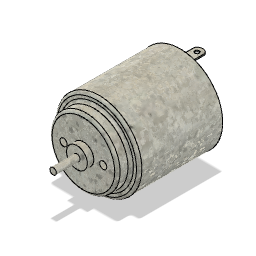
moteur DC (Autodesk Fusion 360 design; units mm, degrees)
Autodesk Fusion 360 part; units mm, degrees
sketch "Esquisse1" plane through (0, 0, 0) normal (0, 0, 1) x (1, 0, 0)
  circle A0 centre (0, 0) radius 2.9
  circle A1 centre (0, 0) radius 9.45
  circle A2 centre (0, 0) radius 11.8
  line L0 (0, 0) -> (-4.5, 0) construction
  circle A3 centre (-5.5, 0.0034) radius 1
  line L1 (-6.5, 0) -> (-4.5, 0)
  line L2 (0, 0) -> (0, 1.3273)
  circle A4 centre (5.5, 0.0034) radius 1
  line L3 (0, 0) -> (0, 8.7) construction
  line L4 (0, 0) -> (0, 8.35) construction
  line L5 (0, 8.35) -> (-1.45, 8.35)
  line L6 (0, 8.7) -> (-1.45, 8.7)
  line L7 (-1.45, 8.7) -> (-1.45, 8.35)
  line L8 (0, 8.7) -> (1.45, 8.7)
  line L9 (0, 8.35) -> (1.45, 8.35)
  line L10 (1.45, 8.7) -> (1.45, 8.35)
  line L11 (0, -8.35) -> (-1.45, -8.35)
  line L12 (0, -8.35) -> (1.45, -8.35)
  line L13 (0, -8.7) -> (1.45, -8.7)
  line L14 (0, -8.7) -> (-1.45, -8.7)
  line L15 (-1.45, -8.7) -> (-1.45, -8.35)
  line L16 (1.45, -8.7) -> (1.45, -8.35)
  circle A5 centre (0, 0) radius 0.9
  dimension "d1" = 5.8
  dimension "d2" = 18.9
  dimension "d3" = 23.6
  dimension "d4" = 4.5
  dimension "d5" = 2
  dimension "d6" = 5.5
  dimension "d7" = 8.7
  dimension "d8" = 8.35
  dimension "d9" = 1.45
  dimension "d10" = 1.45
  dimension "d21" = 1.8
  constraint coincident A0.centre A1.centre
  constraint concentric A1 A2
  constraint horizontal L0
  constraint coincident L0.end A3
  constraint coincident A3 L1.start
  constraint parallel L0 L1
  constraint perpendicular L0 L2
  constraint symmetric A3 L2 A4
  constraint perpendicular L0 L3
  constraint perpendicular L0 L4
  constraint perpendicular L4 L5
  constraint perpendicular L3 L6
  constraint symmetric L6.start L3 L8.start
  constraint symmetric L3 L4.end L5.start
  constraint symmetric L3 L5.end L9.end
  constraint symmetric L3 L6.end L8.end
  constraint symmetric L0 L3.end L13.start
  constraint symmetric L0 L4.end L11.start
  constraint symmetric L0 L5.end L11.end
  constraint symmetric L0 L6.end L14.end
  constraint symmetric L0 L8.end L13.end
  constraint symmetric L0 L9.end L12.end
  constraint concentric A0 A5
  measures "d1" diameter of A0
  measures "d2" diameter of A1
  measures "d3" diameter of A2
  measures "d4" distance of A0.centre L0.end
  measures "d5" diameter of A3
  measures "d6" distance of A0.centre A3.centre
  measures "d7" distance of A0.centre L3.end
  measures "d8" distance of A0.centre L4.end
  measures "d9" distance of L3.end L6.end
  measures "d10" distance of L4.end L5.end
  measures "d21" diameter of A5
extrude "Extrusion1" add sketch "Esquisse1" against normal blind 6.3 contours L5 L6 L7 L8 L9 L10 | L11 L12 L13 L14 L15 L16 makes body 1 at (-0.4833, -8.7, -2.1) makes body 2 at (0.4833, 8.7, -2.1)
extrude "Extrusion2" add sketch "Esquisse1" along normal blind 23.2 separate body contours A2 makes body 3
extrude "Extrusion3" add sketch "Esquisse1" 2 faces at (0.4833, -8.5833, 0) (-0.4833, 8.5833, 0) along normal blind 26.9 contours A1 on bodies 1 2 bodies 1 3 2
extrude "Extrusion4" add sketch "Esquisse1" along normal blind 28.7 and the other way blind 2 separate body contours A0 | A5 makes body 4
extrude "Extrusion5" add sketch "Esquisse1" along normal blind 35.3 contours A5 bodies 4
extrude "Extrusion6" add sketch "Esquisse1" against normal blind 3 contours A5 bodies 4
fillet "Congé1" radius 0.75 3 edges at (-8.8105, -3.4173, 26.9) (-8.8105, 3.4173, 23.2) (-11.0015, -4.2671, 23.2) on bodies 1 3
sketch "Esquisse2" plane through (0, 8.7, 0) normal (0, 1, 0) x (-1, 0, 0)
  line L0 (-1.45, 0) -> (-1.45, -6.3)
  line L1 (-1.45, -6.3) -> (1.45, -6.3)
  line L2 (1.45, -6.3) -> (1.45, 0)
  circle A0 centre (0, -4.7) radius 0.6
  arc A1 (-1.45, -5.3764) -> (1.45, -5.3764) centre (0, -4.7) ccw
  line L3 (1.45, 0) -> (-1.45, 0)
  constraint concentric A0 A1
  constraint tangent L1 A1
  constraint coincident L0 A1.start
  constraint coincident L2 A1.end
extrude "Extrusion7" cut sketch "Esquisse2" against normal blind 20 contours L0 L1 A1 | L1 L2 A1 | A0 bodies 1
sketch "Esquisse3" plane through (0, 0, 0) normal (1, 0, 0) x (0, 0, -1)
equation "d4 = ( 9 / 2 ) * 1 mm"
equation "d7 = 17.4 mm / 2"
equation "d8 = ( 16.7 / 2 ) * 1 mm"
equation "d9 = 2.9 mm / 2"
equation "d10 = ( 2.9 / 2 ) * 1 mm"
equation "d22 = 28.70 mm + 6.6 mm"
